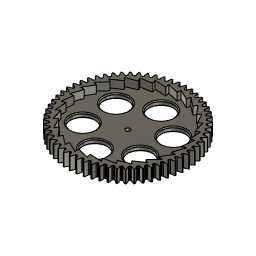
SpringBarrel v2 (Autodesk Fusion 360 design; units mm, degrees)
Autodesk Fusion 360 part; units mm, degrees
sketch "bottom" plane through (0, 0, 0) normal (0, 0, 1) x (1, 0, 0)
  circle A0 centre (0, 0) radius 2.25
  circle A1 centre (0, 0) radius 51
  circle A2 centre (0, 0) radius 55
  line L0 (0, 51) -> (0, 55)
  line L1 (0, 55) -> (10.601, 49.8861)
  line L2 (-11.4351, 53.7981) -> (-0.0026, 51)
  line L3 (-10.6035, 49.8855) -> (-11.4351, 53.7981)
  line L4 (-22.3705, 50.245) -> (-10.606, 49.885)
  line L5 (-20.7436, 46.5908) -> (-22.3705, 50.245)
  line L6 (-32.3282, 44.4959) -> (-20.7459, 46.5898)
  line L7 (-29.977, 41.2599) -> (-32.3282, 44.4959)
  line L8 (-40.873, 36.8022) -> (-29.9791, 41.2583)
  line L9 (-37.9004, 34.1257) -> (-40.873, 36.8022)
  line L10 (-47.6314, 27.5) -> (-37.9021, 34.1237)
  line L11 (-44.1673, 25.5) -> (-47.6314, 27.5)
  line L12 (-52.3081, 16.9959) -> (-44.1686, 25.4978)
  line L13 (-48.5039, 15.7599) -> (-52.3081, 16.9959)
  line L14 (-54.6987, 5.7491) -> (-48.5047, 15.7574)
  line L15 (-50.7206, 5.331) -> (-54.6987, 5.7491)
  line L16 (-54.6987, -5.7491) -> (-50.7209, 5.3284)
  line L17 (-50.7206, -5.331) -> (-54.6987, -5.7491)
  line L18 (-52.3081, -16.9959) -> (-50.7203, -5.3335)
  line L19 (-48.5039, -15.7599) -> (-52.3081, -16.9959)
  line L20 (-47.6314, -27.5) -> (-48.5031, -15.7623)
  line L21 (-44.1673, -25.5) -> (-47.6314, -27.5)
  line L22 (-40.873, -36.8022) -> (-44.166, -25.5022)
  line L23 (-37.9004, -34.1257) -> (-40.873, -36.8022)
  line L24 (-32.3282, -44.4959) -> (-37.8987, -34.1276)
  line L25 (-29.977, -41.2599) -> (-32.3282, -44.4959)
  line L26 (-22.3705, -50.245) -> (-29.975, -41.2614)
  line L27 (-20.7436, -46.5908) -> (-22.3705, -50.245)
  line L28 (-11.4351, -53.7981) -> (-20.7412, -46.5919)
  line L29 (-10.6035, -49.8855) -> (-11.4351, -53.7981)
  line L30 (0, -55) -> (-10.601, -49.8861)
  line L31 (0, -51) -> (0, -55)
  line L32 (11.4351, -53.7981) -> (0.0026, -51)
  line L33 (10.6035, -49.8855) -> (11.4351, -53.7981)
  line L34 (22.3705, -50.245) -> (10.606, -49.885)
  line L35 (20.7436, -46.5908) -> (22.3705, -50.245)
  line L36 (32.3282, -44.4959) -> (20.7459, -46.5898)
  line L37 (29.977, -41.2599) -> (32.3282, -44.4959)
  line L38 (40.873, -36.8022) -> (29.9791, -41.2583)
  line L39 (37.9004, -34.1257) -> (40.873, -36.8022)
  line L40 (47.6314, -27.5) -> (37.9021, -34.1237)
  line L41 (44.1673, -25.5) -> (47.6314, -27.5)
  line L42 (52.3081, -16.9959) -> (44.1686, -25.4978)
  line L43 (48.5039, -15.7599) -> (52.3081, -16.9959)
  line L44 (54.6987, -5.7491) -> (48.5047, -15.7574)
  line L45 (50.7206, -5.331) -> (54.6987, -5.7491)
  line L46 (54.6987, 5.7491) -> (50.7209, -5.3284)
  line L47 (50.7206, 5.331) -> (54.6987, 5.7491)
  line L48 (52.3081, 16.9959) -> (50.7203, 5.3335)
  line L49 (48.5039, 15.7599) -> (52.3081, 16.9959)
  line L50 (47.6314, 27.5) -> (48.5031, 15.7623)
  line L51 (44.1673, 25.5) -> (47.6314, 27.5)
  line L52 (40.873, 36.8022) -> (44.166, 25.5022)
  line L53 (37.9004, 34.1257) -> (40.873, 36.8022)
  line L54 (32.3282, 44.4959) -> (37.8987, 34.1276)
  line L55 (29.977, 41.2599) -> (32.3282, 44.4959)
  line L56 (22.3705, 50.245) -> (29.975, 41.2614)
  line L57 (20.7436, 46.5908) -> (22.3705, 50.245)
  line L58 (11.4351, 53.7981) -> (20.7412, 46.5919)
  line L59 (10.6035, 49.8855) -> (11.4351, 53.7981)
  circle A3 centre (0, 0) radius 62
  circle A4 centre (0, 0) radius 57.5
  line L60 (-0.0026, 51) -> (-0.0026, 34.375) construction
  circle A5 centre (-0.0026, 34.375) radius 12.625
  circle A6 centre (-29.7709, 17.1853) radius 12.625
  circle A7 centre (-29.7683, -17.1897) radius 12.625
  circle A8 centre (0.0026, -34.375) radius 12.625
  circle A9 centre (29.7709, -17.1853) radius 12.625
  circle A10 centre (29.7683, 17.1897) radius 12.625
  line L61 (-1.7477, 61.9761) -> (-1.1479, 61.9901)
  line L62 (-4.0405, 57.3579) -> (1.358, 57.484) construction
  line L63 (-1.4478, 61.9831) -> (0, 0) construction
  arc A11 (-1.7923, 61.9434) -> (-3.2899, 57.883) centre (15.5472, 53.2416) ccw
  arc A12 (-3.9851, 57.3617) -> (-3.2899, 57.883) centre (-4.0405, 58.1598) ccw
  arc A13 (0.5838, 57.9735) -> (-1.1018, 61.9596) centre (-18.0162, 52.4576) ccw
  arc A14 (0.5343, 58.1376) -> (1.3034, 57.4852) centre (1.3206, 58.285) ccw
  arc A15 (-1.1018, 61.9596) -> (-1.1572, 61.9892) centre (-1.1479, 61.9401) ccw
  arc A16 (-1.7383, 61.9756) -> (-1.7923, 61.9434) centre (-1.7454, 61.9261) ccw
  arc A17 (-5.4793, 57.7169) -> (-7.5723, 61.505) centre (-23.4008, 50.2871) ccw
  arc A18 (-9.9592, 56.631) -> (-9.3223, 57.222) centre (-10.0977, 57.4189) ccw
  arc A19 (-8.2573, 61.4168) -> (-9.3223, 57.222) centre (9.8968, 54.5751) ccw
  arc A20 (-8.207, 61.4544) -> (-8.2573, 61.4168) centre (-8.2089, 61.4044) ccw
  line L64 (-8.2164, 61.4539) -> (-7.6213, 61.5305)
  arc A21 (-7.5723, 61.505) -> (-7.6305, 61.5287) centre (-7.6161, 61.4808) ccw
  arc A22 (-5.5457, 57.875) -> (-4.7125, 57.3066) centre (-4.7791, 58.1038) ccw
  arc A23 (-11.4824, 56.828) -> (-13.9599, 60.3765) centre (-28.529, 47.5655) ccw
  arc A24 (-15.8241, 55.2797) -> (-15.2526, 55.9341) centre (-16.0443, 56.0488) ccw
  arc A25 (-14.6319, 60.2172) -> (-15.2526, 55.9341) centre (4.1379, 55.3106) ccw
  arc A26 (-14.5858, 60.2599) -> (-14.6319, 60.2172) centre (-14.5824, 60.21) ccw
  line L65 (-14.5951, 60.2584) -> (-14.0113, 60.3968)
  arc A27 (-13.9599, 60.3765) -> (-14.0202, 60.394) centre (-14.0009, 60.3479) ccw
  arc A28 (-11.5649, 56.9782) -> (-10.6769, 56.5) centre (-10.8264, 57.2859) ccw
  arc A29 (-17.3596, 55.3164) -> (-20.1945, 58.5866) centre (-33.3447, 44.3229) ccw
  arc A30 (-21.5158, 53.3228) -> (-21.0157, 54.0333) centre (-21.8151, 54.0647) ccw
  arc A31 (-20.8461, 58.3579) -> (-21.0157, 54.0333) centre (-1.6663, 55.4401) ccw
  arc A32 (-20.8047, 58.4052) -> (-20.8461, 58.3579) centre (-20.7962, 58.3559) ccw
  line L66 (-20.8138, 58.4027) -> (-20.2477, 58.6014)
  arc A33 (-20.1945, 58.5866) -> (-20.2563, 58.5976) centre (-20.2322, 58.5538) ccw
  arc A34 (-17.4574, 55.4573) -> (-16.5243, 55.0745) centre (-16.7551, 55.8405) ccw
  arc A35 (-23.0466, 53.1988) -> (-26.2078, 56.1547) centre (-37.795, 40.5946) ccw
  arc A36 (-26.9716, 50.7817) -> (-26.5486, 51.5406) centre (-27.3469, 51.4882) ccw
  arc A37 (-26.832, 55.8592) -> (-26.5486, 51.5406) centre (-7.4522, 54.9623) ccw
  arc A38 (-26.7958, 55.9105) -> (-26.832, 55.8592) centre (-26.7821, 55.8624) ccw
  line L67 (-26.8046, 55.9071) -> (-26.2623, 56.1639)
  arc A39 (-26.2078, 56.1547) -> (-26.2705, 56.1593) centre (-26.2419, 56.1182) ccw
  arc A40 (-23.1586, 53.3287) -> (-22.1906, 53.0455) centre (-22.5002, 53.7832) ccw
  arc A41 (-28.4812, 50.4984) -> (-31.934, 53.1076) centre (-41.8313, 36.4216) ccw
  arc A42 (-32.132, 47.6842) -> (-31.7906, 48.4832) centre (-32.5791, 48.3476) ccw
  arc A43 (-32.5239, 52.7484) -> (-31.7906, 48.4832) centre (-13.1565, 53.8822) ccw
  arc A44 (-32.4932, 52.8033) -> (-32.5239, 52.7484) centre (-32.4746, 52.7569) ccw
  line L68 (-32.5016, 52.799) -> (-31.9891, 53.1111)
  arc A45 (-31.934, 53.1076) -> (-31.9968, 53.1056) centre (-31.9641, 53.0677) ccw
  arc A46 (-28.6061, 50.6158) -> (-27.6138, 50.4354) centre (-27.9989, 51.1366) ccw
  arc A47 (-33.6037, 47.2446) -> (-37.3103, 49.4787) centre (-45.4092, 31.8495) ccw
  arc A48 (-36.9404, 44.0643) -> (-36.6844, 44.8945) centre (-37.4543, 44.6773) ccw
  arc A49 (-37.8594, 49.0598) -> (-36.6844, 44.8945) centre (-18.7166, 52.2118) ccw
  arc A50 (-37.8347, 49.1176) -> (-37.8594, 49.0598) centre (-37.8113, 49.0734) ccw
  line L69 (-37.8426, 49.1124) -> (-37.3655, 49.4763)
  arc A51 (-37.3103, 49.4787) -> (-37.3726, 49.4701) centre (-37.3361, 49.4359) ccw
  arc A52 (-33.7402, 47.3484) -> (-32.7345, 47.2727) centre (-33.1907, 47.9298) ccw
  arc A53 (-38.358, 43.4733) -> (-42.2779, 45.3077) centre (-48.4896, 26.9285) ccw
  arc A54 (-41.344, 39.9616) -> (-41.1762, 40.8141) centre (-41.9192, 40.5175) ccw
  arc A55 (-42.7802, 44.8337) -> (-41.1762, 40.8141) centre (-24.0717, 49.9694) ccw
  arc A56 (-42.7616, 44.8937) -> (-42.7802, 44.8337) centre (-42.7337, 44.8522) ccw
  line L70 (-42.7689, 44.8878) -> (-42.3325, 45.2995)
  arc A57 (-42.2779, 45.3077) -> (-42.3389, 45.2926) centre (-42.299, 45.2624) ccw
  arc A58 (-38.5046, 43.5622) -> (-37.4965, 43.592) centre (-38.0189, 44.1979) ccw
  arc A59 (-42.6921, 39.2256) -> (-46.7822, 40.6402) centre (-51.0388, 21.7124) ccw
  arc A60 (-45.2946, 35.421) -> (-45.2168, 36.2864) centre (-45.9248, 35.9138) ccw
  arc A61 (-47.2322, 40.1163) -> (-45.2168, 36.2864) centre (-29.1631, 47.1794) ccw
  arc A62 (-47.22, 40.178) -> (-47.2322, 40.1163) centre (-47.188, 40.1396) ccw
  line L71 (-47.2267, 40.1713) -> (-46.8357, 40.6264)
  arc A63 (-46.7822, 40.6402) -> (-46.8413, 40.6189) centre (-46.7985, 40.593) ccw
  arc A64 (-42.8471, 39.2987) -> (-41.8477, 39.4338) centre (-42.4306, 39.9817) ccw
  arc A65 (-46.5584, 34.5482) -> (-50.774, 35.5275) centre (-53.0287, 16.2585) ccw
  arc A66 (-48.749, 30.4924) -> (-48.7621, 31.3612) centre (-49.4272, 30.9167) ccw
  arc A67 (-51.1668, 34.9594) -> (-48.7621, 31.3612) centre (-33.9349, 43.8726) ccw
  arc A68 (-51.1611, 35.022) -> (-51.1668, 34.9594) centre (-51.1252, 34.9872) ccw
  line L72 (-51.167, 35.0147) -> (-50.8257, 35.5082)
  arc A69 (-50.774, 35.5275) -> (-50.8305, 35.5001) centre (-50.7853, 35.4788) ccw
  arc A70 (-46.7203, 34.6047) -> (-45.7404, 34.8435) centre (-46.3774, 35.3275) ccw
  arc A71 (-49.9146, 29.4923) -> (-54.2095, 30.0256) centre (-54.4377, 10.6264) ccw
  arc A72 (-51.6693, 25.2297) -> (-51.7731, 26.0923) centre (-52.3881, 25.5807) ccw
  arc A73 (-54.5407, 29.4195) -> (-51.7731, 26.0923) centre (-38.335, 40.0851) ccw
  arc A74 (-54.5416, 29.4824) -> (-54.5407, 29.4195) centre (-54.5023, 29.4515) ccw
  line L73 (-54.5467, 29.4745) -> (-54.2589, 30.001)
  arc A75 (-54.2095, 30.0256) -> (-54.2628, 29.9924) centre (-54.2156, 29.976) ccw
  arc A76 (-50.0815, 29.5315) -> (-49.1319, 29.8714) centre (-49.816, 30.2862) ccw
  arc A77 (-52.724, 24.1132) -> (-57.051, 24.1947) centre (-55.2503, 4.8779) ccw
  arc A78 (-54.0234, 19.6906) -> (-54.2169, 20.5376) centre (-54.7751, 19.9646) ccw
  arc A79 (-57.3171, 23.5573) -> (-54.2169, 20.5376) centre (-42.315, 35.8584) ccw
  arc A80 (-57.3246, 23.6197) -> (-57.3171, 23.5573) centre (-57.2822, 23.5931) ccw
  line L74 (-57.3288, 23.6113) -> (-57.0977, 24.165)
  arc A81 (-57.051, 24.1947) -> (-57.1006, 24.1561) centre (-57.052, 24.1447) ccw
  arc A82 (-52.894, 24.1348) -> (-51.9852, 24.5721) centre (-52.7089, 24.9131) ccw
  arc A83 (-54.9556, 18.47) -> (-59.2675, 18.0987) centre (-55.4575, -0.9241) ccw
  arc A84 (-55.7857, 13.9357) -> (-56.0666, 14.7579) centre (-56.5619, 14.1296) ccw
  arc A85 (-59.4656, 17.437) -> (-56.0666, 14.7579) centre (-45.8314, 31.2389) ccw
  arc A86 (-59.4795, 17.4983) -> (-59.4656, 17.437) centre (-59.4346, 17.4763) ccw
  line L75 (-59.4828, 17.4895) -> (-59.3108, 18.0643)
  arc A87 (-59.2675, 18.0987) -> (-59.3128, 18.0551) centre (-59.2632, 18.0488) ccw
  arc A88 (-55.127, 18.4737) -> (-54.2689, 19.0036) centre (-55.0243, 19.267) ccw
  arc A89 (-56.5852, 12.6244) -> (-60.8347, 11.8044) centre (-55.0571, -6.7159) ccw
  arc A90 (-56.9368, 8.0282) -> (-57.3021, 8.8165) centre (-57.729, 8.1399) ccw
  arc A91 (-60.9625, 11.1256) -> (-57.3021, 8.8165) centre (-48.8457, 26.277) ccw
  arc A92 (-60.9827, 11.1851) -> (-60.9625, 11.1256) centre (-60.9358, 11.1679) ccw
  line L76 (-60.9851, 11.176) -> (-60.8741, 11.7657)
  arc A93 (-60.8347, 11.8044) -> (-60.8752, 11.7563) centre (-60.8252, 11.7553) ccw
  arc A94 (-56.7561, 12.6101) -> (-55.958, 13.2268) centre (-56.7368, 13.4099) ccw
  arc A95 (-57.5949, 6.6404) -> (-61.7353, 5.3807) centre (-54.0535, -12.4341) ccw
  arc A96 (-57.4641, 2.0327) -> (-57.9098, 2.7785) centre (-58.2636, 2.061) ccw
  arc A97 (-61.7914, 4.6924) -> (-57.9098, 2.7785) centre (-51.3248, 21.0273) ccw
  arc A98 (-61.8178, 4.7494) -> (-61.7914, 4.6924) centre (-61.7693, 4.7372) ccw
  line L77 (-61.8193, 4.7401) -> (-61.7705, 5.3381)
  arc A99 (-61.7353, 5.3807) -> (-61.7706, 5.3287) centre (-61.7208, 5.3329) ccw
  arc A100 (-57.7633, 6.6084) -> (-57.0341, 7.3051) centre (-57.8277, 7.4058) ccw
  arc A101 (-57.9735, 0.5838) -> (-61.9596, -1.1018) centre (-52.4576, -18.0162) ccw
  arc A102 (-57.3617, -3.9851) -> (-57.883, -3.2899) centre (-58.1598, -4.0405) ccw
  arc A103 (-61.9434, -1.7923) -> (-57.883, -3.2899) centre (-53.2416, 15.5472) ccw
  arc A104 (-61.9756, -1.7383) -> (-61.9434, -1.7923) centre (-61.9261, -1.7454) ccw
  line L78 (-61.9761, -1.7477) -> (-61.9901, -1.1479)
  arc A105 (-61.9596, -1.1018) -> (-61.9892, -1.1572) centre (-61.9401, -1.1479) ccw
  arc A106 (-58.1376, 0.5343) -> (-57.4852, 1.3034) centre (-58.285, 1.3206) ccw
  arc A107 (-57.7169, -5.4793) -> (-61.505, -7.5723) centre (-50.2871, -23.4008) ccw
  arc A108 (-56.631, -9.9592) -> (-57.222, -9.3223) centre (-57.4189, -10.0977) ccw
  arc A109 (-61.4168, -8.2573) -> (-57.222, -9.3223) centre (-54.5751, 9.8968) ccw
  arc A110 (-61.4544, -8.207) -> (-61.4168, -8.2573) centre (-61.4044, -8.2089) ccw
  line L79 (-61.4539, -8.2164) -> (-61.5305, -7.6213)
  arc A111 (-61.505, -7.5723) -> (-61.5287, -7.6305) centre (-61.4808, -7.6161) ccw
  arc A112 (-57.875, -5.5457) -> (-57.3066, -4.7125) centre (-58.1038, -4.7791) ccw
  arc A113 (-56.828, -11.4824) -> (-60.3765, -13.9599) centre (-47.5655, -28.529) ccw
  arc A114 (-55.2797, -15.8241) -> (-55.9341, -15.2526) centre (-56.0488, -16.0443) ccw
  arc A115 (-60.2172, -14.6319) -> (-55.9341, -15.2526) centre (-55.3106, 4.1379) ccw
  arc A116 (-60.2599, -14.5858) -> (-60.2172, -14.6319) centre (-60.21, -14.5824) ccw
  line L80 (-60.2584, -14.5951) -> (-60.3968, -14.0113)
  arc A117 (-60.3765, -13.9599) -> (-60.394, -14.0202) centre (-60.3479, -14.0009) ccw
  arc A118 (-56.9782, -11.5649) -> (-56.5, -10.6769) centre (-57.2859, -10.8264) ccw
  arc A119 (-55.3164, -17.3596) -> (-58.5866, -20.1945) centre (-44.3229, -33.3447) ccw
  arc A120 (-53.3228, -21.5158) -> (-54.0333, -21.0157) centre (-54.0647, -21.8151) ccw
  arc A121 (-58.3579, -20.8461) -> (-54.0333, -21.0157) centre (-55.4401, -1.6663) ccw
  arc A122 (-58.4052, -20.8047) -> (-58.3579, -20.8461) centre (-58.3559, -20.7962) ccw
  line L81 (-58.4027, -20.8138) -> (-58.6014, -20.2477)
  arc A123 (-58.5866, -20.1945) -> (-58.5976, -20.2563) centre (-58.5538, -20.2322) ccw
  arc A124 (-55.4573, -17.4574) -> (-55.0745, -16.5243) centre (-55.8405, -16.7551) ccw
  arc A125 (-53.1988, -23.0466) -> (-56.1547, -26.2078) centre (-40.5946, -37.795) ccw
  arc A126 (-50.7817, -26.9716) -> (-51.5406, -26.5486) centre (-51.4882, -27.3469) ccw
  arc A127 (-55.8592, -26.832) -> (-51.5406, -26.5486) centre (-54.9623, -7.4522) ccw
  arc A128 (-55.9105, -26.7958) -> (-55.8592, -26.832) centre (-55.8624, -26.7821) ccw
  line L82 (-55.9071, -26.8046) -> (-56.1639, -26.2623)
  arc A129 (-56.1547, -26.2078) -> (-56.1593, -26.2705) centre (-56.1182, -26.2419) ccw
  arc A130 (-53.3287, -23.1586) -> (-53.0455, -22.1906) centre (-53.7832, -22.5002) ccw
  arc A131 (-50.4984, -28.4812) -> (-53.1076, -31.934) centre (-36.4216, -41.8313) ccw
  arc A132 (-47.6842, -32.132) -> (-48.4832, -31.7906) centre (-48.3476, -32.5791) ccw
  arc A133 (-52.7484, -32.5239) -> (-48.4832, -31.7906) centre (-53.8822, -13.1565) ccw
  arc A134 (-52.8033, -32.4932) -> (-52.7484, -32.5239) centre (-52.7569, -32.4746) ccw
  line L83 (-52.799, -32.5016) -> (-53.1111, -31.9891)
  arc A135 (-53.1076, -31.934) -> (-53.1056, -31.9968) centre (-53.0677, -31.9641) ccw
  arc A136 (-50.6158, -28.6061) -> (-50.4354, -27.6138) centre (-51.1366, -27.9989) ccw
  arc A137 (-47.2446, -33.6037) -> (-49.4787, -37.3103) centre (-31.8495, -45.4092) ccw
  arc A138 (-44.0643, -36.9404) -> (-44.8945, -36.6844) centre (-44.6773, -37.4543) ccw
  arc A139 (-49.0598, -37.8594) -> (-44.8945, -36.6844) centre (-52.2118, -18.7166) ccw
  arc A140 (-49.1176, -37.8347) -> (-49.0598, -37.8594) centre (-49.0734, -37.8113) ccw
  line L84 (-49.1124, -37.8426) -> (-49.4763, -37.3655)
  arc A141 (-49.4787, -37.3103) -> (-49.4701, -37.3726) centre (-49.4359, -37.3361) ccw
  arc A142 (-47.3484, -33.7402) -> (-47.2727, -32.7345) centre (-47.9298, -33.1907) ccw
  arc A143 (-43.4733, -38.358) -> (-45.3077, -42.2779) centre (-26.9285, -48.4896) ccw
  arc A144 (-39.9616, -41.344) -> (-40.8141, -41.1762) centre (-40.5175, -41.9192) ccw
  arc A145 (-44.8337, -42.7802) -> (-40.8141, -41.1762) centre (-49.9694, -24.0717) ccw
  arc A146 (-44.8937, -42.7616) -> (-44.8337, -42.7802) centre (-44.8522, -42.7337) ccw
  line L85 (-44.8878, -42.7689) -> (-45.2995, -42.3325)
  arc A147 (-45.3077, -42.2779) -> (-45.2926, -42.3389) centre (-45.2624, -42.299) ccw
  arc A148 (-43.5622, -38.5046) -> (-43.592, -37.4965) centre (-44.1979, -38.0189) ccw
  arc A149 (-39.2256, -42.6921) -> (-40.6402, -46.7822) centre (-21.7124, -51.0388) ccw
  arc A150 (-35.421, -45.2946) -> (-36.2864, -45.2168) centre (-35.9138, -45.9248) ccw
  arc A151 (-40.1163, -47.2322) -> (-36.2864, -45.2168) centre (-47.1794, -29.1631) ccw
  arc A152 (-40.178, -47.22) -> (-40.1163, -47.2322) centre (-40.1396, -47.188) ccw
  line L86 (-40.1713, -47.2267) -> (-40.6264, -46.8357)
  arc A153 (-40.6402, -46.7822) -> (-40.6189, -46.8413) centre (-40.593, -46.7985) ccw
  arc A154 (-39.2987, -42.8471) -> (-39.4338, -41.8477) centre (-39.9817, -42.4306) ccw
  arc A155 (-34.5482, -46.5584) -> (-35.5275, -50.774) centre (-16.2585, -53.0287) ccw
  arc A156 (-30.4924, -48.749) -> (-31.3612, -48.7621) centre (-30.9167, -49.4272) ccw
  arc A157 (-34.9594, -51.1668) -> (-31.3612, -48.7621) centre (-43.8726, -33.9349) ccw
  arc A158 (-35.022, -51.1611) -> (-34.9594, -51.1668) centre (-34.9872, -51.1252) ccw
  line L87 (-35.0147, -51.167) -> (-35.5082, -50.8257)
  arc A159 (-35.5275, -50.774) -> (-35.5001, -50.8305) centre (-35.4788, -50.7853) ccw
  arc A160 (-34.6047, -46.7203) -> (-34.8435, -45.7404) centre (-35.3275, -46.3774) ccw
  arc A161 (-29.4923, -49.9146) -> (-30.0256, -54.2095) centre (-10.6264, -54.4377) ccw
  arc A162 (-25.2297, -51.6693) -> (-26.0923, -51.7731) centre (-25.5807, -52.3881) ccw
  arc A163 (-29.4195, -54.5407) -> (-26.0923, -51.7731) centre (-40.0851, -38.335) ccw
  arc A164 (-29.4824, -54.5416) -> (-29.4195, -54.5407) centre (-29.4515, -54.5023) ccw
  line L88 (-29.4745, -54.5467) -> (-30.001, -54.2589)
  arc A165 (-30.0256, -54.2095) -> (-29.9924, -54.2628) centre (-29.976, -54.2156) ccw
  arc A166 (-29.5315, -50.0815) -> (-29.8714, -49.1319) centre (-30.2862, -49.816) ccw
  arc A167 (-24.1132, -52.724) -> (-24.1947, -57.051) centre (-4.8779, -55.2503) ccw
  arc A168 (-19.6906, -54.0234) -> (-20.5376, -54.2169) centre (-19.9646, -54.7751) ccw
  arc A169 (-23.5573, -57.3171) -> (-20.5376, -54.2169) centre (-35.8584, -42.315) ccw
  arc A170 (-23.6197, -57.3246) -> (-23.5573, -57.3171) centre (-23.5931, -57.2822) ccw
  line L89 (-23.6113, -57.3288) -> (-24.165, -57.0977)
  arc A171 (-24.1947, -57.051) -> (-24.1561, -57.1006) centre (-24.1447, -57.052) ccw
  arc A172 (-24.1348, -52.894) -> (-24.5721, -51.9852) centre (-24.9131, -52.7089) ccw
  arc A173 (-18.47, -54.9556) -> (-18.0987, -59.2675) centre (0.9241, -55.4575) ccw
  arc A174 (-13.9357, -55.7857) -> (-14.7579, -56.0666) centre (-14.1296, -56.5619) ccw
  arc A175 (-17.437, -59.4656) -> (-14.7579, -56.0666) centre (-31.2389, -45.8314) ccw
  arc A176 (-17.4983, -59.4795) -> (-17.437, -59.4656) centre (-17.4763, -59.4346) ccw
  line L90 (-17.4895, -59.4828) -> (-18.0643, -59.3108)
  arc A177 (-18.0987, -59.2675) -> (-18.0551, -59.3128) centre (-18.0488, -59.2632) ccw
  arc A178 (-18.4737, -55.127) -> (-19.0036, -54.2689) centre (-19.267, -55.0243) ccw
  arc A179 (-12.6244, -56.5852) -> (-11.8044, -60.8347) centre (6.7159, -55.0571) ccw
  arc A180 (-8.0282, -56.9368) -> (-8.8165, -57.3021) centre (-8.1399, -57.729) ccw
  arc A181 (-11.1256, -60.9625) -> (-8.8165, -57.3021) centre (-26.277, -48.8457) ccw
  arc A182 (-11.1851, -60.9827) -> (-11.1256, -60.9625) centre (-11.1679, -60.9358) ccw
  line L91 (-11.176, -60.9851) -> (-11.7657, -60.8741)
  arc A183 (-11.8044, -60.8347) -> (-11.7563, -60.8752) centre (-11.7553, -60.8252) ccw
  arc A184 (-12.6101, -56.7561) -> (-13.2268, -55.958) centre (-13.4099, -56.7368) ccw
  arc A185 (-6.6404, -57.5949) -> (-5.3807, -61.7353) centre (12.4341, -54.0535) ccw
  arc A186 (-2.0327, -57.4641) -> (-2.7785, -57.9098) centre (-2.061, -58.2636) ccw
  arc A187 (-4.6924, -61.7914) -> (-2.7785, -57.9098) centre (-21.0273, -51.3248) ccw
  arc A188 (-4.7494, -61.8178) -> (-4.6924, -61.7914) centre (-4.7372, -61.7693) ccw
  line L92 (-4.7401, -61.8193) -> (-5.3381, -61.7705)
  arc A189 (-5.3807, -61.7353) -> (-5.3287, -61.7706) centre (-5.3329, -61.7208) ccw
  arc A190 (-6.6084, -57.7633) -> (-7.3051, -57.0341) centre (-7.4058, -57.8277) ccw
  arc A191 (-0.5838, -57.9735) -> (1.1018, -61.9596) centre (18.0162, -52.4576) ccw
  arc A192 (3.9851, -57.3617) -> (3.2899, -57.883) centre (4.0405, -58.1598) ccw
  arc A193 (1.7923, -61.9434) -> (3.2899, -57.883) centre (-15.5472, -53.2416) ccw
  arc A194 (1.7383, -61.9756) -> (1.7923, -61.9434) centre (1.7454, -61.9261) ccw
  line L93 (1.7477, -61.9761) -> (1.1479, -61.9901)
  arc A195 (1.1018, -61.9596) -> (1.1572, -61.9892) centre (1.1479, -61.9401) ccw
  arc A196 (-0.5343, -58.1376) -> (-1.3034, -57.4852) centre (-1.3206, -58.285) ccw
  arc A197 (5.4793, -57.7169) -> (7.5723, -61.505) centre (23.4008, -50.2871) ccw
  arc A198 (9.9592, -56.631) -> (9.3223, -57.222) centre (10.0977, -57.4189) ccw
  arc A199 (8.2573, -61.4168) -> (9.3223, -57.222) centre (-9.8968, -54.5751) ccw
  arc A200 (8.207, -61.4544) -> (8.2573, -61.4168) centre (8.2089, -61.4044) ccw
  line L94 (8.2164, -61.4539) -> (7.6213, -61.5305)
  arc A201 (7.5723, -61.505) -> (7.6305, -61.5287) centre (7.6161, -61.4808) ccw
  arc A202 (5.5457, -57.875) -> (4.7125, -57.3066) centre (4.7791, -58.1038) ccw
  arc A203 (11.4824, -56.828) -> (13.9599, -60.3765) centre (28.529, -47.5655) ccw
  arc A204 (15.8241, -55.2797) -> (15.2526, -55.9341) centre (16.0443, -56.0488) ccw
  arc A205 (14.6319, -60.2172) -> (15.2526, -55.9341) centre (-4.1379, -55.3106) ccw
  arc A206 (14.5858, -60.2599) -> (14.6319, -60.2172) centre (14.5824, -60.21) ccw
  line L95 (14.5951, -60.2584) -> (14.0113, -60.3968)
  arc A207 (13.9599, -60.3765) -> (14.0202, -60.394) centre (14.0009, -60.3479) ccw
  arc A208 (11.5649, -56.9782) -> (10.6769, -56.5) centre (10.8264, -57.2859) ccw
  arc A209 (17.3596, -55.3164) -> (20.1945, -58.5866) centre (33.3447, -44.3229) ccw
  arc A210 (21.5158, -53.3228) -> (21.0157, -54.0333) centre (21.8151, -54.0647) ccw
  arc A211 (20.8461, -58.3579) -> (21.0157, -54.0333) centre (1.6663, -55.4401) ccw
  arc A212 (20.8047, -58.4052) -> (20.8461, -58.3579) centre (20.7962, -58.3559) ccw
  line L96 (20.8138, -58.4027) -> (20.2477, -58.6014)
  arc A213 (20.1945, -58.5866) -> (20.2563, -58.5976) centre (20.2322, -58.5538) ccw
  arc A214 (17.4574, -55.4573) -> (16.5243, -55.0745) centre (16.7551, -55.8405) ccw
  arc A215 (23.0466, -53.1988) -> (26.2078, -56.1547) centre (37.795, -40.5946) ccw
  arc A216 (26.9716, -50.7817) -> (26.5486, -51.5406) centre (27.3469, -51.4882) ccw
  arc A217 (26.832, -55.8592) -> (26.5486, -51.5406) centre (7.4522, -54.9623) ccw
  arc A218 (26.7958, -55.9105) -> (26.832, -55.8592) centre (26.7821, -55.8624) ccw
  line L97 (26.8046, -55.9071) -> (26.2623, -56.1639)
  arc A219 (26.2078, -56.1547) -> (26.2705, -56.1593) centre (26.2419, -56.1182) ccw
  arc A220 (23.1586, -53.3287) -> (22.1906, -53.0455) centre (22.5002, -53.7832) ccw
  arc A221 (28.4812, -50.4984) -> (31.934, -53.1076) centre (41.8313, -36.4216) ccw
  arc A222 (32.132, -47.6842) -> (31.7906, -48.4832) centre (32.5791, -48.3476) ccw
  arc A223 (32.5239, -52.7484) -> (31.7906, -48.4832) centre (13.1565, -53.8822) ccw
  arc A224 (32.4932, -52.8033) -> (32.5239, -52.7484) centre (32.4746, -52.7569) ccw
  line L98 (32.5016, -52.799) -> (31.9891, -53.1111)
  arc A225 (31.934, -53.1076) -> (31.9968, -53.1056) centre (31.9641, -53.0677) ccw
  arc A226 (28.6061, -50.6158) -> (27.6138, -50.4354) centre (27.9989, -51.1366) ccw
  arc A227 (33.6037, -47.2446) -> (37.3103, -49.4787) centre (45.4092, -31.8495) ccw
  arc A228 (36.9404, -44.0643) -> (36.6844, -44.8945) centre (37.4543, -44.6773) ccw
  arc A229 (37.8594, -49.0598) -> (36.6844, -44.8945) centre (18.7166, -52.2118) ccw
  arc A230 (37.8347, -49.1176) -> (37.8594, -49.0598) centre (37.8113, -49.0734) ccw
  line L99 (37.8426, -49.1124) -> (37.3655, -49.4763)
  arc A231 (37.3103, -49.4787) -> (37.3726, -49.4701) centre (37.3361, -49.4359) ccw
  arc A232 (33.7402, -47.3484) -> (32.7345, -47.2727) centre (33.1907, -47.9298) ccw
  arc A233 (38.358, -43.4733) -> (42.2779, -45.3077) centre (48.4896, -26.9285) ccw
  arc A234 (41.344, -39.9616) -> (41.1762, -40.8141) centre (41.9192, -40.5175) ccw
  arc A235 (42.7802, -44.8337) -> (41.1762, -40.8141) centre (24.0717, -49.9694) ccw
  arc A236 (42.7616, -44.8937) -> (42.7802, -44.8337) centre (42.7337, -44.8522) ccw
  line L100 (42.7689, -44.8878) -> (42.3325, -45.2995)
  arc A237 (42.2779, -45.3077) -> (42.3389, -45.2926) centre (42.299, -45.2624) ccw
  arc A238 (38.5046, -43.5622) -> (37.4965, -43.592) centre (38.0189, -44.1979) ccw
  arc A239 (42.6921, -39.2256) -> (46.7822, -40.6402) centre (51.0388, -21.7124) ccw
  arc A240 (45.2946, -35.421) -> (45.2168, -36.2864) centre (45.9248, -35.9138) ccw
  arc A241 (47.2322, -40.1163) -> (45.2168, -36.2864) centre (29.1631, -47.1794) ccw
  arc A242 (47.22, -40.178) -> (47.2322, -40.1163) centre (47.188, -40.1396) ccw
  line L101 (47.2267, -40.1713) -> (46.8357, -40.6264)
  arc A243 (46.7822, -40.6402) -> (46.8413, -40.6189) centre (46.7985, -40.593) ccw
  arc A244 (42.8471, -39.2987) -> (41.8477, -39.4338) centre (42.4306, -39.9817) ccw
  arc A245 (46.5584, -34.5482) -> (50.774, -35.5275) centre (53.0287, -16.2585) ccw
  arc A246 (48.749, -30.4924) -> (48.7621, -31.3612) centre (49.4272, -30.9167) ccw
  arc A247 (51.1668, -34.9594) -> (48.7621, -31.3612) centre (33.9349, -43.8726) ccw
  arc A248 (51.1611, -35.022) -> (51.1668, -34.9594) centre (51.1252, -34.9872) ccw
  line L102 (51.167, -35.0147) -> (50.8257, -35.5082)
  arc A249 (50.774, -35.5275) -> (50.8305, -35.5001) centre (50.7853, -35.4788) ccw
  arc A250 (46.7203, -34.6047) -> (45.7404, -34.8435) centre (46.3774, -35.3275) ccw
  arc A251 (49.9146, -29.4923) -> (54.2095, -30.0256) centre (54.4377, -10.6264) ccw
  arc A252 (51.6693, -25.2297) -> (51.7731, -26.0923) centre (52.3881, -25.5807) ccw
  arc A253 (54.5407, -29.4195) -> (51.7731, -26.0923) centre (38.335, -40.0851) ccw
  arc A254 (54.5416, -29.4824) -> (54.5407, -29.4195) centre (54.5023, -29.4515) ccw
  line L103 (54.5467, -29.4745) -> (54.2589, -30.001)
  arc A255 (54.2095, -30.0256) -> (54.2628, -29.9924) centre (54.2156, -29.976) ccw
  arc A256 (50.0815, -29.5315) -> (49.1319, -29.8714) centre (49.816, -30.2862) ccw
  arc A257 (52.724, -24.1132) -> (57.051, -24.1947) centre (55.2503, -4.8779) ccw
  arc A258 (54.0234, -19.6906) -> (54.2169, -20.5376) centre (54.7751, -19.9646) ccw
  arc A259 (57.3171, -23.5573) -> (54.2169, -20.5376) centre (42.315, -35.8584) ccw
  arc A260 (57.3246, -23.6197) -> (57.3171, -23.5573) centre (57.2822, -23.5931) ccw
  line L104 (57.3288, -23.6113) -> (57.0977, -24.165)
  arc A261 (57.051, -24.1947) -> (57.1006, -24.1561) centre (57.052, -24.1447) ccw
  arc A262 (52.894, -24.1348) -> (51.9852, -24.5721) centre (52.7089, -24.9131) ccw
  arc A263 (54.9556, -18.47) -> (59.2675, -18.0987) centre (55.4575, 0.9241) ccw
  arc A264 (55.7857, -13.9357) -> (56.0666, -14.7579) centre (56.5619, -14.1296) ccw
  arc A265 (59.4656, -17.437) -> (56.0666, -14.7579) centre (45.8314, -31.2389) ccw
  arc A266 (59.4795, -17.4983) -> (59.4656, -17.437) centre (59.4346, -17.4763) ccw
  line L105 (59.4828, -17.4895) -> (59.3108, -18.0643)
  arc A267 (59.2675, -18.0987) -> (59.3128, -18.0551) centre (59.2632, -18.0488) ccw
  arc A268 (55.127, -18.4737) -> (54.2689, -19.0036) centre (55.0243, -19.267) ccw
  arc A269 (56.5852, -12.6244) -> (60.8347, -11.8044) centre (55.0571, 6.7159) ccw
  arc A270 (56.9368, -8.0282) -> (57.3021, -8.8165) centre (57.729, -8.1399) ccw
  arc A271 (60.9625, -11.1256) -> (57.3021, -8.8165) centre (48.8457, -26.277) ccw
  arc A272 (60.9827, -11.1851) -> (60.9625, -11.1256) centre (60.9358, -11.1679) ccw
  line L106 (60.9851, -11.176) -> (60.8741, -11.7657)
  arc A273 (60.8347, -11.8044) -> (60.8752, -11.7563) centre (60.8252, -11.7553) ccw
  arc A274 (56.7561, -12.6101) -> (55.958, -13.2268) centre (56.7368, -13.4099) ccw
  arc A275 (57.5949, -6.6404) -> (61.7353, -5.3807) centre (54.0535, 12.4341) ccw
  arc A276 (57.4641, -2.0327) -> (57.9098, -2.7785) centre (58.2636, -2.061) ccw
  arc A277 (61.7914, -4.6924) -> (57.9098, -2.7785) centre (51.3248, -21.0273) ccw
  arc A278 (61.8178, -4.7494) -> (61.7914, -4.6924) centre (61.7693, -4.7372) ccw
  line L107 (61.8193, -4.7401) -> (61.7705, -5.3381)
  arc A279 (61.7353, -5.3807) -> (61.7706, -5.3287) centre (61.7208, -5.3329) ccw
  arc A280 (57.7633, -6.6084) -> (57.0341, -7.3051) centre (57.8277, -7.4058) ccw
  arc A281 (57.9735, -0.5838) -> (61.9596, 1.1018) centre (52.4576, 18.0162) ccw
  arc A282 (57.3617, 3.9851) -> (57.883, 3.2899) centre (58.1598, 4.0405) ccw
  arc A283 (61.9434, 1.7923) -> (57.883, 3.2899) centre (53.2416, -15.5472) ccw
  arc A284 (61.9756, 1.7383) -> (61.9434, 1.7923) centre (61.9261, 1.7454) ccw
  line L108 (61.9761, 1.7477) -> (61.9901, 1.1479)
  arc A285 (61.9596, 1.1018) -> (61.9892, 1.1572) centre (61.9401, 1.1479) ccw
  arc A286 (58.1376, -0.5343) -> (57.4852, -1.3034) centre (58.285, -1.3206) ccw
  arc A287 (57.7169, 5.4793) -> (61.505, 7.5723) centre (50.2871, 23.4008) ccw
  arc A288 (56.631, 9.9592) -> (57.222, 9.3223) centre (57.4189, 10.0977) ccw
  arc A289 (61.4168, 8.2573) -> (57.222, 9.3223) centre (54.5751, -9.8968) ccw
  arc A290 (61.4544, 8.207) -> (61.4168, 8.2573) centre (61.4044, 8.2089) ccw
  line L109 (61.4539, 8.2164) -> (61.5305, 7.6213)
  arc A291 (61.505, 7.5723) -> (61.5287, 7.6305) centre (61.4808, 7.6161) ccw
  arc A292 (57.875, 5.5457) -> (57.3066, 4.7125) centre (58.1038, 4.7791) ccw
  arc A293 (56.828, 11.4824) -> (60.3765, 13.9599) centre (47.5655, 28.529) ccw
  arc A294 (55.2797, 15.8241) -> (55.9341, 15.2526) centre (56.0488, 16.0443) ccw
  arc A295 (60.2172, 14.6319) -> (55.9341, 15.2526) centre (55.3106, -4.1379) ccw
  arc A296 (60.2599, 14.5858) -> (60.2172, 14.6319) centre (60.21, 14.5824) ccw
  line L110 (60.2584, 14.5951) -> (60.3968, 14.0113)
  arc A297 (60.3765, 13.9599) -> (60.394, 14.0202) centre (60.3479, 14.0009) ccw
  arc A298 (56.9782, 11.5649) -> (56.5, 10.6769) centre (57.2859, 10.8264) ccw
  arc A299 (55.3164, 17.3596) -> (58.5866, 20.1945) centre (44.3229, 33.3447) ccw
  arc A300 (53.3228, 21.5158) -> (54.0333, 21.0157) centre (54.0647, 21.8151) ccw
  arc A301 (58.3579, 20.8461) -> (54.0333, 21.0157) centre (55.4401, 1.6663) ccw
  arc A302 (58.4052, 20.8047) -> (58.3579, 20.8461) centre (58.3559, 20.7962) ccw
  line L111 (58.4027, 20.8138) -> (58.6014, 20.2477)
  arc A303 (58.5866, 20.1945) -> (58.5976, 20.2563) centre (58.5538, 20.2322) ccw
  arc A304 (55.4573, 17.4574) -> (55.0745, 16.5243) centre (55.8405, 16.7551) ccw
  arc A305 (53.1988, 23.0466) -> (56.1547, 26.2078) centre (40.5946, 37.795) ccw
  arc A306 (50.7817, 26.9716) -> (51.5406, 26.5486) centre (51.4882, 27.3469) ccw
  arc A307 (55.8592, 26.832) -> (51.5406, 26.5486) centre (54.9623, 7.4522) ccw
  arc A308 (55.9105, 26.7958) -> (55.8592, 26.832) centre (55.8624, 26.7821) ccw
  line L112 (55.9071, 26.8046) -> (56.1639, 26.2623)
  arc A309 (56.1547, 26.2078) -> (56.1593, 26.2705) centre (56.1182, 26.2419) ccw
  arc A310 (53.3287, 23.1586) -> (53.0455, 22.1906) centre (53.7832, 22.5002) ccw
  arc A311 (50.4984, 28.4812) -> (53.1076, 31.934) centre (36.4216, 41.8313) ccw
  arc A312 (47.6842, 32.132) -> (48.4832, 31.7906) centre (48.3476, 32.5791) ccw
  arc A313 (52.7484, 32.5239) -> (48.4832, 31.7906) centre (53.8822, 13.1565) ccw
  arc A314 (52.8033, 32.4932) -> (52.7484, 32.5239) centre (52.7569, 32.4746) ccw
  line L113 (52.799, 32.5016) -> (53.1111, 31.9891)
  arc A315 (53.1076, 31.934) -> (53.1056, 31.9968) centre (53.0677, 31.9641) ccw
  arc A316 (50.6158, 28.6061) -> (50.4354, 27.6138) centre (51.1366, 27.9989) ccw
  arc A317 (47.2446, 33.6037) -> (49.4787, 37.3103) centre (31.8495, 45.4092) ccw
  arc A318 (44.0643, 36.9404) -> (44.8945, 36.6844) centre (44.6773, 37.4543) ccw
  arc A319 (49.0598, 37.8594) -> (44.8945, 36.6844) centre (52.2118, 18.7166) ccw
  arc A320 (49.1176, 37.8347) -> (49.0598, 37.8594) centre (49.0734, 37.8113) ccw
  line L114 (49.1124, 37.8426) -> (49.4763, 37.3655)
  arc A321 (49.4787, 37.3103) -> (49.4701, 37.3726) centre (49.4359, 37.3361) ccw
  arc A322 (47.3484, 33.7402) -> (47.2727, 32.7345) centre (47.9298, 33.1907) ccw
  arc A323 (43.4733, 38.358) -> (45.3077, 42.2779) centre (26.9285, 48.4896) ccw
  arc A324 (39.9616, 41.344) -> (40.8141, 41.1762) centre (40.5175, 41.9192) ccw
  arc A325 (44.8337, 42.7802) -> (40.8141, 41.1762) centre (49.9694, 24.0717) ccw
  arc A326 (44.8937, 42.7616) -> (44.8337, 42.7802) centre (44.8522, 42.7337) ccw
  line L115 (44.8878, 42.7689) -> (45.2995, 42.3325)
  arc A327 (45.3077, 42.2779) -> (45.2926, 42.3389) centre (45.2624, 42.299) ccw
  arc A328 (43.5622, 38.5046) -> (43.592, 37.4965) centre (44.1979, 38.0189) ccw
  arc A329 (39.2256, 42.6921) -> (40.6402, 46.7822) centre (21.7124, 51.0388) ccw
  arc A330 (35.421, 45.2946) -> (36.2864, 45.2168) centre (35.9138, 45.9248) ccw
  arc A331 (40.1163, 47.2322) -> (36.2864, 45.2168) centre (47.1794, 29.1631) ccw
  arc A332 (40.178, 47.22) -> (40.1163, 47.2322) centre (40.1396, 47.188) ccw
  line L116 (40.1713, 47.2267) -> (40.6264, 46.8357)
  arc A333 (40.6402, 46.7822) -> (40.6189, 46.8413) centre (40.593, 46.7985) ccw
  arc A334 (39.2987, 42.8471) -> (39.4338, 41.8477) centre (39.9817, 42.4306) ccw
  arc A335 (34.5482, 46.5584) -> (35.5275, 50.774) centre (16.2585, 53.0287) ccw
  arc A336 (30.4924, 48.749) -> (31.3612, 48.7621) centre (30.9167, 49.4272) ccw
  arc A337 (34.9594, 51.1668) -> (31.3612, 48.7621) centre (43.8726, 33.9349) ccw
  arc A338 (35.022, 51.1611) -> (34.9594, 51.1668) centre (34.9872, 51.1252) ccw
  line L117 (35.0147, 51.167) -> (35.5082, 50.8257)
  arc A339 (35.5275, 50.774) -> (35.5001, 50.8305) centre (35.4788, 50.7853) ccw
  arc A340 (34.6047, 46.7203) -> (34.8435, 45.7404) centre (35.3275, 46.3774) ccw
  arc A341 (29.4923, 49.9146) -> (30.0256, 54.2095) centre (10.6264, 54.4377) ccw
  arc A342 (25.2297, 51.6693) -> (26.0923, 51.7731) centre (25.5807, 52.3881) ccw
  arc A343 (29.4195, 54.5407) -> (26.0923, 51.7731) centre (40.0851, 38.335) ccw
  arc A344 (29.4824, 54.5416) -> (29.4195, 54.5407) centre (29.4515, 54.5023) ccw
  line L118 (29.4745, 54.5467) -> (30.001, 54.2589)
  arc A345 (30.0256, 54.2095) -> (29.9924, 54.2628) centre (29.976, 54.2156) ccw
  arc A346 (29.5315, 50.0815) -> (29.8714, 49.1319) centre (30.2862, 49.816) ccw
  arc A347 (24.1132, 52.724) -> (24.1947, 57.051) centre (4.8779, 55.2503) ccw
  arc A348 (19.6906, 54.0234) -> (20.5376, 54.2169) centre (19.9646, 54.7751) ccw
  arc A349 (23.5573, 57.3171) -> (20.5376, 54.2169) centre (35.8584, 42.315) ccw
  arc A350 (23.6197, 57.3246) -> (23.5573, 57.3171) centre (23.5931, 57.2822) ccw
  line L119 (23.6113, 57.3288) -> (24.165, 57.0977)
  arc A351 (24.1947, 57.051) -> (24.1561, 57.1006) centre (24.1447, 57.052) ccw
  arc A352 (24.1348, 52.894) -> (24.5721, 51.9852) centre (24.9131, 52.7089) ccw
  arc A353 (18.47, 54.9556) -> (18.0987, 59.2675) centre (-0.9241, 55.4575) ccw
  arc A354 (13.9357, 55.7857) -> (14.7579, 56.0666) centre (14.1296, 56.5619) ccw
  arc A355 (17.437, 59.4656) -> (14.7579, 56.0666) centre (31.2389, 45.8314) ccw
  arc A356 (17.4983, 59.4795) -> (17.437, 59.4656) centre (17.4763, 59.4346) ccw
  line L120 (17.4895, 59.4828) -> (18.0643, 59.3108)
  arc A357 (18.0987, 59.2675) -> (18.0551, 59.3128) centre (18.0488, 59.2632) ccw
  arc A358 (18.4737, 55.127) -> (19.0036, 54.2689) centre (19.267, 55.0243) ccw
  arc A359 (12.6244, 56.5852) -> (11.8044, 60.8347) centre (-6.7159, 55.0571) ccw
  arc A360 (8.0282, 56.9368) -> (8.8165, 57.3021) centre (8.1399, 57.729) ccw
  arc A361 (11.1256, 60.9625) -> (8.8165, 57.3021) centre (26.277, 48.8457) ccw
  arc A362 (11.1851, 60.9827) -> (11.1256, 60.9625) centre (11.1679, 60.9358) ccw
  line L121 (11.176, 60.9851) -> (11.7657, 60.8741)
  arc A363 (11.8044, 60.8347) -> (11.7563, 60.8752) centre (11.7553, 60.8252) ccw
  arc A364 (12.6101, 56.7561) -> (13.2268, 55.958) centre (13.4099, 56.7368) ccw
  arc A365 (6.6404, 57.5949) -> (5.3807, 61.7353) centre (-12.4341, 54.0535) ccw
  arc A366 (2.0327, 57.4641) -> (2.7785, 57.9098) centre (2.061, 58.2636) ccw
  arc A367 (4.6924, 61.7914) -> (2.7785, 57.9098) centre (21.0273, 51.3248) ccw
  arc A368 (4.7494, 61.8178) -> (4.6924, 61.7914) centre (4.7372, 61.7693) ccw
  line L122 (4.7401, 61.8193) -> (5.3381, 61.7705)
  arc A369 (5.3807, 61.7353) -> (5.3287, 61.7706) centre (5.3329, 61.7208) ccw
  arc A370 (6.6084, 57.7633) -> (7.3051, 57.0341) centre (7.4058, 57.8277) ccw
  point P0 (0.8876, 57.816)
  point P1 (-3.5861, 57.7115)
  dimension "d1" = 4.5
  dimension "d2" = 102
  dimension "d3" = 110
  dimension "d4" = 11.77
  dimension "d6" = 360
  dimension "d7" = 124
  dimension "d8" = 115
  dimension "d9" = 16.625
  dimension "d10" = 25.25
  dimension "d12" = 360
  dimension "d13" = 0.6
  dimension "d14" = 0.1
  dimension "d16" = 5.4
  dimension "d17" = 1.6
  dimension "d19" = 360
  constraint coincident A0.centre A1.centre
  constraint concentric A0 A1
  constraint coincident A1 L0.start
  constraint coincident A2 L0.end
  constraint vertical L0
  constraint coincident A1 L1.end
  constraint concentric A0 A3
  constraint concentric A2 A4
  constraint vertical L60
  constraint coincident L60.end A5.centre
  constraint tangent L61 A15
  constraint vertical L61.end A15.centre
  constraint midpoint L61 L63.start
  constraint symmetric L62.start L62.end L63
  constraint coincident A4 L62.end
  constraint tangent A4 A12
  constraint symmetric L63 A15 A16
  constraint symmetric L63 A12 A14
  constraint symmetric L61.start L61.end L63
  constraint symmetric L63 P0 P1
  constraint vertical L62.start A12.centre
  constraint coincident A3 L63.start
  constraint coincident A4 A12.start
  constraint symmetric L63 A11.end A13.start
  constraint symmetric L63 A11.start A13.end
  constraint symmetric L63 A11 A13
  constraint coincident A4 A14.end
  constraint coincident A13 A14.start
  constraint coincident A3 A15.end
  constraint coincident A3 A16.start
  measures "d1" diameter of A0
  measures "d2" diameter of A1
  measures "d3" diameter of A2
  measures "d4" distance of L0.end L1.end
  measures "d7" diameter of A3
  measures "d8" diameter of A4
  measures "d9" distance of L2.end L60.end
  measures "d10" diameter of A5
  measures "d13" distance of L61.start L61.end
  measures "d14" diameter of A15
  measures "d16" distance of L62.start L62.end
  measures "d17" diameter of A12
extrude "Extrude1" add sketch "bottom" along normal blind 5 contours A1 L0 L1 makes body 1
extrude "Extrude2" add sketch "bottom" along normal blind 5 contours A1 bodies 1
pattern_circular "C-Pattern1" count 30 over 360 about axis through (0, 0, 0) along (0, 0, 1) of "Extrude1"
extrude "Extrude3" add sketch "bottom" along normal blind 13 contours A1 A2 L0 L2 bodies 1
pattern_circular "C-Pattern2" count 30 over 360 about axis through (0, 0, 0) along (0, 0, 1) of "Extrude3"
extrude "Extrude4" add sketch "bottom" along normal blind 13 separate body contours A3 A4 L61 A11 A12 A13 A14 A15 A16 makes body 2
pattern_circular "C-Pattern3" count 60 over 360 about axis through (0, 0, 0) along (0, 0, 1) of "Extrude4" makes body 3 at (-5.2983, 57.2554, 4.3333) makes body 4 at (-11.2541, 56.3879, 4.3333) makes body 5 at (-17.0866, 54.9026, 4.3333) makes body 6 at (-22.7318, 52.8158, 4.3333) makes body 7 at (-28.1281, 50.1504, 4.3333) makes body 8 at (-33.2161, 46.9355, 4.3333) makes body 9 at (-37.9403, 43.2063, 4.3333) makes body 10 at (-42.2487, 39.0038, 8.6667) makes body 11 at (-46.0943, 34.3739, 4.3333) makes body 12 at (-49.4348, 29.3675, 4.3333) makes body 13 at (-52.2338, 24.0392, 8.6667) makes body 14 at (-54.4604, 18.4476, 4.3333) makes body 15 at (-56.0904, 12.6539, 4.3333) makes body 16 at (-57.1058, 6.7216, 4.3333) makes body 17 at (-57.4955, 0.7156, 4.3333) makes body 18 at (-57.2554, -5.2983, 4.3333) makes body 19 at (-56.3879, -11.2541, 4.3333) makes body 20 at (-54.9026, -17.0866, 4.3333) makes body 21 at (-52.8158, -22.7318, 4.3333) makes body 22 at (-50.1504, -28.1281, 4.3333) makes body 23 at (-46.9355, -33.2161, 4.3333) makes body 24 at (-43.2063, -37.9403, 4.3333) makes body 25 at (-39.0038, -42.2487, 8.6667) makes body 26 at (-34.3739, -46.0943, 4.3333) makes body 27 at (-29.3675, -49.4348, 4.3333) makes body 28 at (-24.0392, -52.2338, 8.6667) makes body 29 at (-18.4476, -54.4604, 4.3333) makes body 30 at (-12.6539, -56.0904, 4.3333) makes body 31 at (-6.7216, -57.1058, 4.3333) makes body 32 at (-0.7156, -57.4955, 4.3333) makes body 33 at (5.2983, -57.2554, 4.3333) makes body 34 at (11.2541, -56.3879, 4.3333) makes body 35 at (17.0866, -54.9026, 4.3333) makes body 36 at (22.7318, -52.8158, 4.3333) makes body 37 at (28.1281, -50.1504, 4.3333) makes body 38 at (33.2161, -46.9355, 4.3333) makes body 39 at (37.9403, -43.2063, 4.3333) makes body 40 at (42.2487, -39.0038, 4.3333) makes body 41 at (46.0943, -34.3739, 4.3333) makes body 42 at (49.4348, -29.3675, 4.3333) makes body 43 at (52.2338, -24.0392, 8.6667) makes body 44 at (54.4604, -18.4476, 4.3333) makes body 45 at (56.0904, -12.6539, 4.3333) makes body 46 at (57.1058, -6.7216, 4.3333) makes body 47 at (57.4955, -0.7156, 4.3333) makes body 48 at (57.2554, 5.2983, 4.3333) makes body 49 at (56.3879, 11.2541, 4.3333) makes body 50 at (54.9026, 17.0866, 4.3333) makes body 51 at (52.8158, 22.7318, 4.3333) makes body 52 at (50.1504, 28.1281, 4.3333) makes body 53 at (46.9355, 33.2161, 4.3333) makes body 54 at (43.2063, 37.9403, 4.3333) makes body 55 at (39.0038, 42.2487, 8.6667) makes body 56 at (34.3739, 46.0943, 4.3333) makes body 57 at (29.3675, 49.4348, 4.3333) makes body 58 at (24.0392, 52.2338, 8.6667) makes body 59 at (18.4476, 54.4604, 4.3333) makes body 60 at (12.6539, 56.0904, 4.3333) makes body 61 at (6.7216, 57.1058, 4.3333)
extrude "Extrude5" add sketch "bottom" along normal blind 13 contours A4 bodies 1 2 3 4 5 6 7 8 9 10 11 12 13 14 15 16 17 18 19 20 21 22 23 24 25 26 27 28 29 30 31 32 33 34 35 36 37 38 39 40 41 42 43 44 45 46 47 48 49 50 51 52 53 54 55 56 57 58 59 60 61
fillet "Fillet1" radius 1 2 edges at (17.9977, 21.7551, 5) (17.9977, 21.7551, 0) on bodies 1
fillet "Fillet2" radius 1 5 edges at (-41.539, -12.6243, 5) (-11.7681, -29.8096, 5) (-41.5415, 21.7507, 5) (-11.7732, 38.9404, 5) (18.0003, -12.6199, 5) on bodies 1
fillet "Fillet3" radius 1 5 edges at (18.0003, -12.6199, 0) (-11.7681, -29.8096, 0) (-41.539, -12.6243, 0) (-41.5415, 21.7507, 0) (-11.7732, 38.9404, 0) on bodies 1
equation "d9 = ( ( 25.25 / 2 ) * 1 mm ) + 4 mm"
named bodies: "SpringBarrel"
